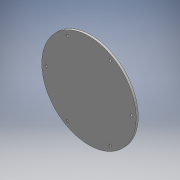
# Autodesk Inventor part: Top
Saved by Autodesk Inventor 2016 (Build 200138000, 138)
## iProperties
Created: 2016-03-11
Part Number: Top
Material: Generic
Document SubType Name: Modeling
Designer: s_sud
Density: 1 g/cm^3
Appearance: Default
Author: s_sud
Autodesk Inventor part; units mm, degrees
ref_plane "YZ Plane" through (0, 0, 0) normal (1, 0, 0) x (0, 1, 0)
ref_plane "XZ Plane" through (0, 0, 0) normal (0, 1, 0) x (-1, 0, 0)
ref_plane "XY Plane" through (0, 0, 0) normal (0, 0, 1) x (1, 0, 0)
sketch "Sketch1" plane through (0, 0, 0) normal (0, 1, 0) x (-1, 0, 0)
  circle A0 centre (0, 0) radius 66.5
  dimension "d0" = 133
  constraints: 1 centre point, 1 coincident
  measures "d0" diameter of A0
extrude "Extrusion1" add sketch "Sketch1" along normal blind 3
sketch "Sketch2" plane through (0, 3, 0) normal (0, 1, 0) x (1, 0, 0)
  circle A0 centre (0, 0) radius 55
  circle A1 centre (-60, 0) radius 1.5
  circle A2 centre (-30, -51.9615) radius 1.5
  circle A3 centre (30, -51.9615) radius 1.5
  circle A4 centre (60, 0) radius 1.5
  circle A5 centre (30, 51.9615) radius 1.5
  circle A6 centre (-30, 51.9615) radius 1.5
  dimension "d3" = 110
  dimension "d4" = 3
  dimension "d5" = 60
  dimension "d8" = 360
  constraints: 7 centre point, 1 coincident, 13 other
  measures "d3" diameter of A0
  measures "d4" diameter of A1
  measures "d5" distance of point (0, 0) A1.centre
extrude "Extrusion2" cut sketch "Sketch2" against normal blind 3 contours A1 | A2 | A3 | A4 | A5 | A6
body "Solid1"
